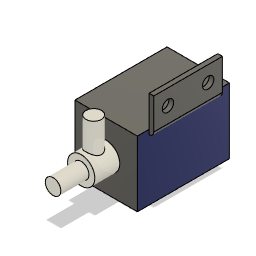
Solenoid+Assembly (Autodesk Fusion 360 archive; units mm, degrees)
design "Solenoid Valve"
Autodesk Fusion 360 part; units mm, degrees
sketch "Sketch1" plane through (0, 0, 0) normal (0, 0, 1) x (1, 0, 0)
  line L0 (0, 0) -> (20, 0)
  line L1 (20, 0) -> (20, 21)
  line L2 (20, 21) -> (0, 21)
  line L3 (0, 21) -> (0, 0)
  dimension "d1" = 20
  dimension "d2" = 21
  constraint horizontal L0
  constraint vertical L1
  constraint horizontal L2
  constraint vertical L3
  constraint coincident L0.start L3.end
  measures "d1" distance of L1.end L2.end
  measures "d2" distance of L0.start L2.end
extrude "Extrude1" add sketch "Sketch1" along normal blind 29.5 makes body 1
sketch "Sketch2" plane through (20, 0, 0) normal (1, 0, 0) x (0, 0, -1)
  line L0 (0, 0) -> (0, 21)
  line L1 (0, 21) -> (-29.5, 21)
  line L2 (-29.5, 21) -> (-29.5, 0)
  line L3 (-29.5, 0) -> (0, 0)
  line L4 (-25.75, 21) -> (-3.75, 21)
  line L5 (-3.75, 21) -> (-3.75, 31)
  line L6 (-3.75, 31) -> (-25.75, 31)
  line L7 (-25.75, 31) -> (-25.75, 21)
  line L8 (0, 0) -> (0, 21)
  line L9 (0, 0) -> (-29.5, 0)
  circle A0 centre (-21.2, 26) radius 1.825
  circle A1 centre (-8.3, 26) radius 1.825
  line L10 (-8.3, 26) -> (-21.2, 26) construction
  point P0 (-14.75, 0)
  point P1 (-14.75, 31)
  point P2 (-14.75, 26)
  point P3 (-3.75, 26)
  dimension "d5" = 22
  dimension "d6" = 10
  dimension "d7" = 3.65
  dimension "d8" = 3.65
  dimension "d9" = 12.9
  constraint horizontal L4
  constraint vertical L5
  constraint horizontal L6
  constraint vertical L7
  constraint coincident L1 L4.start
  constraint midpoint L3 P0
  constraint midpoint L6 P1
  constraint vertical P0 P1
  constraint horizontal A0.centre A1.centre
  constraint coincident A1.centre L10.start
  constraint coincident A0.centre L10.end
  constraint midpoint L10 P2
  constraint vertical P1 P2
  constraint midpoint L5 P3
  constraint horizontal A1.centre P3
  measures "d5" distance of L5.end L6.end
  measures "d6" distance of L4 L6
  measures "d7" diameter of A0
  measures "d8" diameter of A1
  measures "d9" distance of A0.centre A1.centre
extrude "Extrude2" add sketch "Sketch2" along normal blind 1.5 separate body contours L1 L4 L5 L6 L7 makes body 2
extrude "Extrude3" add 1 faces at (20.5, 21, 11.0833) along direction (0, -1, 0) blind 1.5 on bodies 2 bodies 2 1
fillet "Fillet1" radius 1.5 1 edges at (21.5, 19.5, 14.75) on bodies 2
sketch "Sketch3" plane through (0, 0, 29.5) normal (0, 0, 1) x (1, 0, 0)
  line L0 (0, 21) -> (0, 0)
  line L1 (0, 0) -> (20, 0)
  line L2 (20, 0) -> (20, 21)
  line L3 (20, 21) -> (0, 21)
  circle A0 centre (10, 10.5) radius 4.375
  point P0 (20, 10.5)
  point P1 (10, 0)
  dimension "d15" = 8.75
  constraint midpoint L2 P0
  constraint midpoint L1 P1
  constraint horizontal A0.centre P0
  constraint vertical A0.centre P1
  measures "d15" diameter of A0
extrude "Extrude4" add sketch "Sketch3" along normal blind 8 contours A0 bodies 2
sketch "Sketch4" plane through (0, 0, 37.5) normal (0, 0, 1) x (1, 0, 0)
  circle A0 centre (10, 10.5) radius 4.375
  circle A1 centre (10, 10.5) radius 2.5
  dimension "d18" = 5
  constraint concentric A0 A1
  measures "d18" diameter of A1
extrude "Extrude5" add sketch "Sketch4" along normal blind 9 contours A1 bodies 2
ref_plane "WorkPlane1" through (10, 10.5, 14.75) normal (0, 1, 0) x (-1, 0, 0)
sketch "Sketch5" plane through (10, 10.5, 14.75) normal (0, 1, 0) x (1, 0, 0)
  line L0 (-4.375, -22.75) -> (4.375, -22.75)
  circle A0 centre (0, -18.75) radius 2.5
  point P0 (0, -22.75)
  dimension "d21" = 5
  dimension "d22" = 4
  constraint midpoint L0 P0
  constraint vertical A0.centre P0
  measures "d21" diameter of A0
  measures "d22" vertical distance of A0.centre P0
extrude "Extrude6" add sketch "Sketch5" along normal blind 13.375 bodies 2
equation "d8 = d7"
equation "d23 = ( 8.75 / 2 ) * 1 mm + 9 mm"
